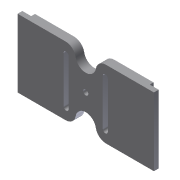
# Autodesk Inventor part: JointB2
Saved by Autodesk Inventor 2013 (Build 170138000, 138)
## iProperties
Created: 2012-10-15
Part Number: JointB2
Document SubType Name: Modeling
Designer: JohnHenry
Density: 1 g/cm^3
Material: 一般
Mass: 12.9856 g
Surface Area: 74.9607 cm^2
Volume: 12.9856 cm^3
Author: JohnHenry
Autodesk Inventor part; units mm, degrees
ref_plane "YZ Plane" through (0, 0, 0) normal (1, 0, 0) x (0, 1, 0)
ref_plane "XZ Plane" through (0, 0, 0) normal (0, 1, 0) x (-1, 0, 0)
ref_plane "XY Plane" through (0, 0, 0) normal (0, 0, 1) x (1, 0, 0)
sketch "スケッチ1" plane through (0, 0, 0) normal (0, 0, 1) x (1, 0, 0)
  line L0 (-40, 2.4068) -> (40, 2.4068)
  line L1 (40, 2.4068) -> (40, -2.5932)
  line L2 (40, -2.5932) -> (-40, -2.5932)
  line L3 (-40, -2.5932) -> (-40, 2.4068)
  point P0 (0, 0)
  dimension "d0" = 5
  dimension "d2" = 80
  dimension "d3" = 40
  constraints: 8 end point, 2 parallel, 1 horizontal, 1 perpendicular
  measures "d0" distance of L0.end L1.end
  measures "d2" distance of L1.end L2.end
  measures "d3" distance from line of L1 point (0, 0)
extrude "押し出し1" add sketch "スケッチ1" along normal blind 40
sketch "スケッチ2" plane through (-40, 2.4068, 0) normal (0, 1, 0) x (1, 0, 0)
  line L0 (0, -40) -> (80, -40) projected
  line L1 (80, 0) -> (80, -40) projected
  line L2 (0, 0) -> (5.2, 0)
  line L3 (5.2, 0) -> (5.2, -40)
  line L4 (5.2, -40) -> (0, -40)
  line L5 (0, -40) -> (0, 0)
  line L6 (80, 0) -> (74.8, 0)
  line L7 (74.8, 0) -> (74.8, -40)
  line L8 (74.8, -40) -> (80, -40)
  line L9 (80, -40) -> (80, 0)
  point P0 (40, 0)
  dimension "d6" = 5.2
  dimension "d7" = 5.2
  constraints: 16 end point, 4 parallel, 2 horizontal, 2 perpendicular, 2 point on line
  measures "d6" distance of L2.start L2.end
  measures "d7" distance between parallel lines of L1 L7
extrude "押し出し2" cut sketch "スケッチ2" against normal blind 2.2
sketch "スケッチ4" plane through (-34.8, 2.4068, 0) normal (0, 1, 0) x (1, 0, 0)
  line L0 (69.6, -40) -> (69.6, 0) projected
  line L1 (0, 0) -> (69.6, 0) projected
  point P0 (34.8, 0)
  point P1 (34.8, -20)
  dimension "d19" = 20
  dimension "d20" = 34.8
  measures "d19" distance from line of point (34.8, -20) L1
  measures "d20" distance from line of L0 point (34.8, -20)
hole "Hole2" at (0, 2.4068, 20) direction (0, -1, 0) diameter 3 end through all
sketch "スケッチ5" plane through (-40, -2.5932, 0) normal (0, -1, 0) x (1, 0, 0)
  circle A0 centre (40, 20) radius 1.5 projected
  line L0 (80, 40) -> (0, 40) projected
  line L1 (80, 0) -> (0, 0) projected
  line L2 (27, 35) -> (30, 35)
  line L3 (30, 35) -> (30, 5)
  line L4 (30, 5) -> (27, 5)
  line L5 (27, 5) -> (27, 35)
  line L6 (50, 35) -> (53, 35)
  line L7 (53, 35) -> (53, 5)
  line L8 (53, 5) -> (50, 5)
  line L9 (50, 5) -> (50, 35)
  point P0 (40, 0)
  dimension "d28" = 3
  dimension "d29" = 3
  dimension "d30" = 5
  dimension "d31" = 5
  dimension "d32" = 5
  dimension "d33" = 5
  dimension "d34" = 10
  dimension "d35" = 10
  constraints: 16 end point, 4 parallel, 2 horizontal, 2 perpendicular
  measures "d28" distance of L2.start L2.end
  measures "d29" distance of L6.start L6.end
  measures "d30" distance between parallel lines of L6 L0
  measures "d31" distance between parallel lines of L1 L8
  measures "d32" distance between parallel lines of L2 L0
  measures "d33" distance between parallel lines of L1 L4
  measures "d34" distance from line of L3 A0.centre
  measures "d35" distance from line of L9 A0.centre
extrude "押し出し3" cut sketch "スケッチ5" against normal through all contours L2 L3 L4 L5 | L6 L7 L8 L9
fillet "フィレット1" radius 1.5 8 edges at (10, -0.0932, 35) (13, -0.0932, 35) (13, -0.0932, 5) (10, -0.0932, 5) (-10, -0.0932, 35) (-13, -0.0932, 35) (-10, -0.0932, 5) (-13, -0.0932, 5)
sketch "スケッチ6" plane through (-40, -2.5932, 0) normal (0, -1, 0) x (1, 0, 0)
  circle A0 centre (40, 20) radius 1.5 projected
  line L0 (80, 40) -> (0, 40) projected
  line L1 (80, 0) -> (0, 0) projected
  line L2 (34, 40) -> (46, 40)
  line L3 (46, 40) -> (46, 30)
  line L4 (46, 30) -> (34, 30)
  line L5 (34, 30) -> (34, 40)
  line L6 (34, 0) -> (46, 0)
  line L7 (46, 0) -> (46, 10)
  line L8 (46, 10) -> (34, 10)
  line L9 (34, 10) -> (34, 0)
  point P0 (40, 0)
  dimension "d39" = 12
  dimension "d40" = 12
  dimension "d41" = 6
  dimension "d42" = 6
  dimension "d43" = 10
  dimension "d44" = 10
  constraints: 16 end point, 4 parallel, 2 horizontal, 2 perpendicular, 2 point on line
  measures "d39" distance of L3.end L4.end
  measures "d40" distance of L7.end L8.end
  measures "d41" distance from line of L7 point (40, 0)
  measures "d42" distance from line of L3 A0.centre
  measures "d43" distance of L2.end L3.end
  measures "d44" distance of L6.end L7.end
extrude "押し出し4" cut sketch "スケッチ6" against normal through all contours L3 L4 L5 L0 | L1 L9 L8 L7
fillet "フィレット2" radius 6 4 edges at (-6, -0.0932, 30) (6, -0.0932, 30) (6, -0.0932, 10) (-6, -0.0932, 10)
fillet "フィレット3" radius 6 4 edges at (-6, -0.0932, 40) (6, -0.0932, 40) (6, -0.0932, 0) (-6, -0.0932, 0)
equation "\"d3\" = 0.5 * d2"
equation "\"d7\" = d6"
equation "\"d29\" = d28"
equation "\"d31\" = d30"
equation "\"d32\" = d30"
equation "\"d33\" = d30"
equation "\"d35\" = d34"
equation "\"d39\" = d40"
equation "\"d41\" = 0.5 * d40"
equation "\"d42\" = d41"
equation "\"d44\" = d43"
equation "\"d47\" = 0.5 * d40"
equation "\"d48\" = 0.5 * d40"
